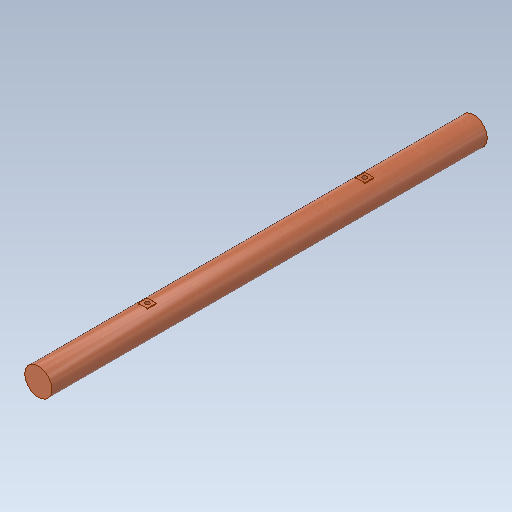
# Autodesk Inventor part: CrossMember-6-Feet
Saved by Autodesk Inventor 2020.1 (Build 241239000, 239)
## iProperties
Created: 2018-11-23
Part Number: CrossMember-6-Feet
Material: Wood (Walnut)
Document SubType Name: Modeling
Designer: steele
Density: 0.55 g/cm^3
Appearance: Walnut - Natural Polished
Author: steele
Autodesk Inventor part; units mm, degrees
ref_plane "YZ Plane" through (0, 0, 0) normal (1, 0, 0) x (0, 1, 0)
ref_plane "XY Plane" through (0, 0, 0) normal (0, 0, 1) x (1, 0, 0)
sketch "Sketch1" plane through (0, 0, 0) normal (0, 0, 1) x (1, 0, 0)
  circle A0 centre (0, 0) radius 76.2
  dimension "d0" = 152.4
  constraints: 1 centre point, 1 coincident
  measures "d0" diameter of A0
extrude "Extrusion1" add sketch "Sketch1" along normal mid plane 2438.4
ref_plane "Work Plane2" through (0, 76.2, 0) normal (0, 1, 0) x (-1, 0, 0)
sketch "Sketch4" plane through (0, 76.2, 0) normal (0, 1, 0) x (-1, 0, 0)
  line L0 (25.4, 635) -> (25.4, 584.2)
  line L1 (25.4, 584.2) -> (-25.4, 584.2)
  line L2 (-25.4, 584.2) -> (-25.4, 635)
  line L3 (-25.4, 635) -> (25.4, 635)
  line L4 (25.4, 635) -> (-25.4, 584.2) construction
  line L5 (25.4, 584.2) -> (-25.4, 635) construction
  line L6 (76.2, 1219.2) -> (-76.2, 1219.2) projected
  point P0 (0, 0)
  point P1 (0, 609.6)
  dimension "d17" = 50.8
  dimension "d19" = 609.6
  constraints: 12 end point, 2 midpoint, 2 parallel, 2 perpendicular, 1 vertical
  measures "d17" distance of L0.start L0.end
  measures "d19" distance from line of point (0, 609.6) L6
extrude "Extrusion3" add sketch "Sketch4" against normal blind 25.4
mirror "Mirror1" about plane through (0, 0, 0) normal (0, 0, 1) of "Extrusion3"
sketch "Sketch5" plane through (0, 76.2, 0) normal (0, 1, 0) x (1, 0, 0)
  line L0 (76.2, 1219.2) -> (-76.2, 1219.2) projected
  line L1 (-76.2, -1219.2) -> (76.2, -1219.2) projected
  point P0 (0, 0)
  point P1 (0, -609.6)
  point P2 (0, 609.6)
  dimension "d22" = 609.6
  dimension "d23" = 609.6
  measures "d22" distance from line of point (0, 609.6) L0
  measures "d23" distance from line of point (0, -609.6) L1
hole "Hole2" at (0, 76.2, 609.6) at (0, 76.2, -609.6) direction (0, -1, 0) diameter 25.4 end through all
body "Solid1"
